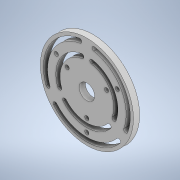
# Autodesk Inventor part: WorkTriangleDisk
Saved by Autodesk Inventor 2021 (Build 250183000, 183)
## iProperties
Created: 2022-09-09
Part Number: WorkTriangleDisk
Material: Generic
Document SubType Name: Modeling
Designer: szucs
Density: 1 g/cm^3
Appearance: Default
Author: szucs
Autodesk Inventor part; units mm, degrees
ref_plane "YZ Plane" through (0, 0, 0) normal (1, 0, 0) x (0, 1, 0)
ref_plane "XZ Plane" through (0, 0, 0) normal (0, 1, 0) x (-1, 0, 0)
ref_plane "XY Plane" through (0, 0, 0) normal (0, 0, 1) x (1, 0, 0)
sketch "Sketch1" plane through (0, 0, 0) normal (0, 0, 1) x (1, 0, 0)
  line L0 (0, 63) -> (0, -63) projected
  line L1 (-63, 0) -> (63, 0) projected
  circle A0 centre (0, 0) radius 45
  dimension "d0" = 90
  constraints: 1 centre point, 1 coincident
  measures "d0" diameter of A0
extrude "Extrusion1" add sketch "Sketch1" along normal blind 6
sketch "Sketch2" plane through (0, 0, 6) normal (0, 0, 1) x (1, 0, 0)
  circle A0 centre (0, 0) radius 7.5
  circle A1 centre (0, 0) radius 45 projected
  line L0 (0, 63) -> (0, -63) projected
  line L1 (-63, 0) -> (63, 0) projected
  arc A2 (-21.4492, -17.9981) -> (21.4492, -17.9981) centre (0, 0) ccw construction
  arc A3 (-22.9813, -19.2836) -> (22.9813, -19.2836) centre (0, 0) ccw
  arc A4 (-19.9172, -16.7125) -> (19.9172, -16.7125) centre (0, 0) ccw
  arc A5 (-19.9172, -16.7125) -> (-22.9813, -19.2836) centre (-21.4492, -17.9981) ccw
  arc A6 (22.9813, -19.2836) -> (19.9172, -16.7125) centre (21.4492, -17.9981) ccw
  line L2 (0, 0) -> (21.4492, -17.9981) construction
  line L3 (0, 0) -> (-21.4492, -17.9981) construction
  arc A7 (-30.6418, -25.7115) -> (30.6418, -25.7115) centre (0, 0) ccw construction
  arc A8 (-32.1739, -26.9971) -> (32.1739, -26.9971) centre (0, 0) ccw
  arc A9 (-29.1097, -24.4259) -> (29.1097, -24.4259) centre (0, 0) ccw
  arc A10 (-29.1097, -24.4259) -> (-32.1739, -26.9971) centre (-30.6418, -25.7115) ccw
  arc A11 (32.1739, -26.9971) -> (29.1097, -24.4259) centre (30.6418, -25.7115) ccw
  line L4 (0, 0) -> (30.6418, -25.7115) construction
  line L5 (0, 0) -> (-30.6418, -25.7115) construction
  circle A12 centre (0, -34) radius 2
  circle A13 centre (0, -22) radius 2
  dimension "d3" = 15
  dimension "d35" = 100
  dimension "d36" = 4
  dimension "d37" = 28
  dimension "d38" = 100
  dimension "d39" = 4
  dimension "d40" = 12
  dimension "d41" = 4
  dimension "d42" = 4
  dimension "d43" = 22
  dimension "d44" = 34
  constraints: 20 point on circle, 13 centre point, 8 end point, 8 tangent, 3 coincident, 2 point on line, 2 symmetric about line
  measures "d3" diameter of A0
  measures "d35" angle of L3 L2
  measures "d36" diameter of A6
  measures "d37" distance of point (0, 0) L3.end
  measures "d38" angle of L5 L4
  measures "d39" diameter of A11
  measures "d40" distance of L5.end L3.end
  measures "d41" diameter of A12
  measures "d42" diameter of A13
  measures "d43" distance of A0.centre A13.centre
  measures "d44" distance of point (0, 0) A12.centre
extrude "Extrusion2" cut sketch "Sketch2" against normal through all contours L1 L0 A0 | A0 L0 L1 | L0 L1 A0 | A0 L1 L0 | A13 L0 | L0 A13 | A8 A10 A9 L0 | L0 A9 A11 A8 | A4 A6 A3 L0 | L0 A3 A5 A4 | A12 L0 | L0 A12
pattern_circular "Circular Pattern2" count 3 over 360 about axis through (0, 0, 6) along (0, 0, -1) of "Extrusion2"
body "Solid1"
